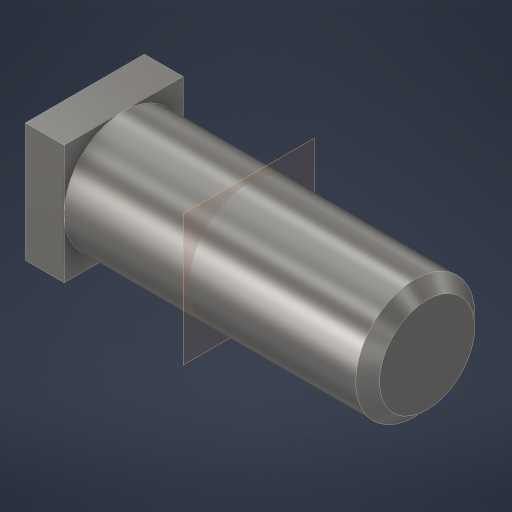
# Autodesk Inventor part: Welle Querrolle Quad
Saved by Autodesk Inventor 2024.1 (Build 281209000, 209)
## iProperties
Part Number: Welle Querrolle Quad
Material: Stahl, Kohlenstoff
Document SubType Name: Modeling
Designer: rYan
Density: 7.85 g/cm^3
Appearance: Halbpoliert
Mass: 0.145715 g
Surface Area: 0.418736 cm^2
Volume: 0.0185624 cm^3
Author: rYan
Autodesk Inventor part; units mm, degrees
ref_plane "XZ Plane" through (0, 0, 0) normal (0, 1, 0) x (-1, 0, 0)
ref_plane "XY Plane" through (0, 0, 0) normal (0, 0, 1) x (1, 0, 0)
sketch "Skizze1" plane through (0, 0, 0) normal (0, 0, 1) x (1, 0, 0)
  line L0 (-2.1, 0) -> (2.8, 0)
  line L1 (2.8, 0) -> (2.8, 1)
  line L2 (2.8, 1) -> (-2.1, 1)
  line L3 (-2.1, 1) -> (-2.1, 0)
  line L4 (0, 1.2) -> (0, -0.2) construction
  line L5 (2.8, 1) -> (3, 0.8)
  line L6 (3, 0.8) -> (3, 0)
  line L7 (3, 0) -> (2.8, 0)
  point P0 (0, 0)
  dimension "d0" = 2
  dimension "d5" = 2.8
  dimension "d8" = 2.1
  dimension "d13" = 45
  dimension "d14" = 0.2
  constraints: 14 end point, 3 perpendicular, 1 horizontal, 1 parallel, 1 point on line, 1 vertical
  measures "d0" diameter of L2 L0
  measures "d5" distance from line of L1.end L4
  measures "d8" distance from line of L2.end L4
  measures "d13" angle of L1 L5
  measures "d14" distance between parallel lines of L1 L6
revolve "Umdrehung1" add sketch "Skizze1" angle 360 about axis through (-2.1, 0, 0) along (1, 0, 0)
sketch "Skizze2" plane through (-2.1, 0, 0) normal (-1, 0, 0) x (0, 0, 1)
  line L0 (-1, -1) -> (1, -1)
  line L1 (1, -1) -> (1, 1)
  line L2 (1, 1) -> (-1, 1)
  line L3 (-1, 1) -> (-1, -1)
  line L4 (-1, -1) -> (1, 1) construction
  line L5 (1, -1) -> (-1, 1) construction
  point P0 (0, 0)
  dimension "d9" = 2
  dimension "d10" = 2
  constraints: 12 end point, 2 midpoint, 2 parallel, 1 horizontal, 1 perpendicular
  measures "d9" distance of L0.end L1.end
  measures "d10" distance of L1.end L2.end
extrude "Extrusion1" add sketch "Skizze2" along normal blind 0.65
sketch "Skizze3" plane through (-2.75, 0, 0) normal (-1, 0, 0) x (0, 0, 1)
  circle A0 centre (0, 0) radius 1.3
  circle A1 centre (0, 0) radius 1.5
  dimension "d15" = 2.6
  dimension "d16" = 3
  constraints: 2 centre point, 2 coincident
  measures "d15" diameter of A0
  measures "d16" diameter of A1
extrude "Extrusion2" [suppressed]
equation "\"d10\" = d9"
